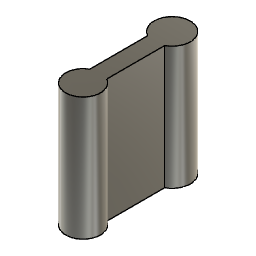
hinge (Autodesk Fusion 360 design; units mm, degrees)
Autodesk Fusion 360 part; units mm, degrees
sketch "Sketch1" plane through (0, 0, 0) normal (0, 0, 1) x (1, 0, 0)
  circle A0 centre (0, 0) radius 2.4
  line L0 (-1.175, 2.0927) -> (-1.175, 10.0927)
  line L1 (1.175, 2.0927) -> (1.175, 10.0927)
  circle A1 centre (0, 12.2994) radius 2.5
  dimension "d1" = 4.8
  dimension "d3" = 2.35
  dimension "d4" = 1.175
  dimension "d5" = 5
  dimension "d6" = 8
  dimension "d7" = 8
  constraint coincident A0.centre origin
  constraint coincident A0 L0.start
  constraint vertical L0
  constraint coincident A0 L1.start
  constraint parallel L0 L1
  constraint coincident L0.end A1
  constraint coincident L1.end A1
  measures "d1" diameter of A0
  measures "d3" distance of L0 L1
  measures "d4" distance of A0.centre L1
  measures "d5" diameter of A1
  measures "d6" distance of L1.start L1.end
  measures "d7" distance of L0.start L0.end
extrude "Extrude1" add sketch "Sketch1" along normal blind 17
